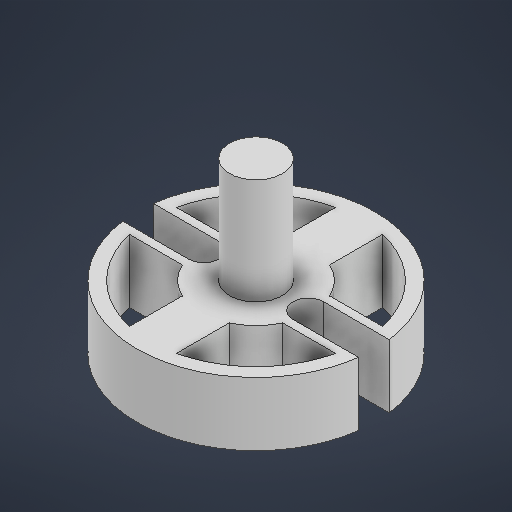
# Autodesk Inventor part: intermo
Saved by Autodesk Inventor 2025.3 (Build 293356000, 356)
## iProperties
Created: 2025-10-02
Part Number: intermo
Material: Generic
Document SubType Name: Modeling
Designer: sophi
Density: 1 g/cm^3
Appearance: Default
Author: sophi
Autodesk Inventor part; units mm, degrees
ref_plane "YZ Plane" through (0, 0, 0) normal (1, 0, 0) x (0, 1, 0)
ref_plane "XZ Plane" through (0, 0, 0) normal (0, 1, 0) x (-1, 0, 0)
ref_plane "XY Plane" through (0, 0, 0) normal (0, 0, 1) x (1, 0, 0)
sketch "Sketch1" plane through (0, 0, 0) normal (0, 1, 0) x (-1, 0, 0)
  circle A0 centre (0, 0) radius 22.5
  circle A1 centre (0, 0) radius 5
  line L0 (19.5029, -4.4313) -> (9.5029, -4.4313)
  line L1 (4.4313, -9.5029) -> (4.4313, -19.5029)
  line L2 (0, 27.7106) -> (0, -38.967) construction
  line L3 (22.5481, 0) -> (-22.5481, 0) construction
  arc A2 (4.4313, -19.5029) -> (19.5029, -4.4313) centre (0, 0) ccw
  arc A3 (4.4313, -9.5029) -> (9.5029, -4.4313) centre (0, 0) ccw
  arc A4 (19.5029, 4.4313) -> (4.4313, 19.5029) centre (0, 0) ccw
  line L4 (4.4313, 19.5029) -> (4.4313, 9.5029)
  arc A5 (9.5029, 4.4313) -> (4.4313, 9.5029) centre (0, 0) ccw
  line L5 (9.5029, 4.4313) -> (19.5029, 4.4313)
  arc A6 (-4.4313, 19.5029) -> (-19.5029, 4.4313) centre (0, 0) ccw
  line L6 (-19.5029, 4.4313) -> (-9.5029, 4.4313)
  arc A7 (-4.4313, 9.5029) -> (-9.5029, 4.4313) centre (0, 0) ccw
  line L7 (-4.4313, 9.5029) -> (-4.4313, 19.5029)
  arc A8 (-19.5029, -4.4313) -> (-4.4313, -19.5029) centre (0, 0) ccw
  line L8 (-4.4313, -19.5029) -> (-4.4313, -9.5029)
  arc A9 (-9.5029, -4.4313) -> (-4.4313, -9.5029) centre (0, 0) ccw
  line L9 (-9.5029, -4.4313) -> (-19.5029, -4.4313)
  dimension "d0" = 45
  dimension "d1" = 10
  dimension "d30" = 10
  dimension "d31" = 40
  dimension "d32" = 20
  dimension "d35" = 360
  constraints: 20 end point, 16 point on circle, 10 centre point, 2 coincident, 2 concentric, 2 horizontal, 2 midpoint, 2 parallel, 2 point on line, 2 vertical, 1 perpendicular, 41 other
  measures "d0" diameter of A0
  measures "d1" diameter of A1
  measures "d30" distance of L0.start L0.end
  measures "d32" radius of A2
extrude "Extrusion1" add sketch "Sketch1" along normal blind 12
sketch "Sketch2" plane through (0, 12, 0) normal (0, 1, 0) x (1, 0, 0)
  line L0 (0, -38.1392) -> (0, 29.2755) construction
  line L1 (-24.9, 0) -> (-9.9, 0) construction
  line L2 (-24.9, -2.9) -> (-9.9, -2.9)
  line L3 (-9.9, 2.9) -> (-24.9, 2.9)
  arc A0 (-24.9, 2.9) -> (-24.9, -2.9) centre (-24.9, 0) ccw
  arc A1 (-9.9, -2.9) -> (-9.9, 2.9) centre (-9.9, 0) ccw
  line L4 (-28.2416, 0) -> (26.6331, 0) construction
  line L5 (24.9, -2.9) -> (9.9, -2.9)
  line L6 (9.9, 2.9) -> (24.9, 2.9)
  arc A2 (24.9, -2.9) -> (24.9, 2.9) centre (24.9, 0) ccw
  arc A3 (9.9, 2.9) -> (9.9, -2.9) centre (9.9, 0) ccw
  point P0 (0, 0)
  point P1 (0, 0)
  point P2 (-17.4, 0)
  point P3 (-7, 0)
  dimension "d49" = 5.8
  dimension "d50" = 7
  dimension "d51" = 15
  constraints: 16 end point, 9 point on circle, 6 symmetric about line, 4 centre point, 4 point on line, 4 tangent, 2 horizontal, 1 midpoint, 1 parallel, 1 vertical, 2 other
  measures "d49" diameter of A1
  measures "d50" distance of point (0, 0) point (-7, 0)
  measures "d51" distance of L3.start L3.end
extrude "Extrusion2" cut sketch "Sketch2" against normal blind 12
ref_plane "Work Plane3" through (22.3123, 12, 2.9) normal (-1, 0, 0) x (0, -1, 0)
sketch "Sketch4" plane through (22.3123, 12, 2.9) normal (-1, 0, 0) x (0, -1, 0)
  line L0 (0, -5.8) -> (12, -5.8) projected
  line L1 (12, 0) -> (0, 0) projected
  line L2 (12, 0) -> (12, -5.8) projected
  line L3 (0, -5.8) -> (0, 0) projected
  circle A0 centre (6, -2.9) radius 1.9
  point P0 (12, -2.9)
  dimension "d52" = 3.8
  dimension "d53" = 6
  dimension "d54" = 2.9
  constraints: 1 centre point
  measures "d52" diameter of A0
  measures "d53" distance from line of L3 A0.centre
  measures "d54" distance from line of L0 A0.centre
extrude "Extrusion4" cut sketch "Sketch4" along normal up to surface contours A0 round surface about axis through (-9.9, 12, 0) along (0, -1, 0) radius 2.9 far side no
ref_plane "Work Plane4" through (0, 12, 0) normal (0, 1, 0) x (1, 0, 0)
sketch "Sketch6" plane through (0, 12, 0) normal (0, 1, 0) x (1, 0, 0)
  circle A0 centre (0, 0) radius 5 projected
  circle A1 centre (0, 0) radius 6.5
  circle A2 centre (0, 0) radius 5
  dimension "d58" = 13
  constraints: 3 concentric, 2 centre point
  measures "d58" diameter of A1
extrude "Extrusion5" add sketch "Sketch6" along normal blind 20 and the other way blind 4 contours A0
body "Solid1"
